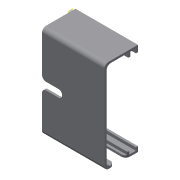
# Autodesk Inventor part: 09_Lid_Electronics
Saved by Autodesk Inventor 2019.4 (Build 234330000, 330)
## iProperties
Created: 2021-03-22
Part Number: 09_Lid_Electronics
Material: Generic
Document SubType Name: Modeling
Designer: diederichbenedict
Density: 1 g/cm^3
Appearance: Default
Author: diederichbenedict
Autodesk Inventor part; units mm, degrees
ref_plane "YZ Plane" through (0, 0, 0) normal (1, 0, 0) x (0, 1, 0)
ref_plane "XZ Plane" through (0, 0, 0) normal (0, 1, 0) x (-1, 0, 0)
ref_plane "Work Plane1" through (-120.5, -62.5, -4) normal (-1, 0, 0) x (0, 1, 0)
sketch "Sketch1" plane through (-120.5, -62.5, -4) normal (-1, 0, 0) x (0, 1, 0)
  line L0 (125, 2) -> (125, -4) projected
  line L1 (0, 2) -> (125, 2) projected
  line L2 (0, 2) -> (0, -4) projected
  line L3 (125, -4) -> (0, -4) projected
  line L4 (129, 6) -> (126, 6)
  line L5 (126, 6) -> (126, -42)
  line L6 (126, -42) -> (129, -42)
  line L7 (129, -42) -> (129, 6)
  line L8 (126, 6) -> (119.9159, 6)
  line L9 (119.9159, 6) -> (119.9159, 3)
  line L10 (119.9159, 3) -> (126, 3)
  line L11 (126, 3) -> (126, 6)
  line L12 (126, -5) -> (119.9159, -5)
  line L13 (119.9159, -5) -> (119.9159, -8)
  line L14 (119.9159, -8) -> (126, -8)
  line L15 (126, -8) -> (126, -5)
  line L16 (126, -42) -> (-4, -42)
  line L17 (-4, -42) -> (-4, -39)
  line L18 (-4, -39) -> (126, -39)
  line L19 (126, -39) -> (126, -42)
  line L20 (-4, -39) -> (-1, -39)
  line L21 (-1, -39) -> (-1, 6)
  line L22 (-1, 6) -> (-4, 6)
  line L23 (-4, 6) -> (-4, -39)
  line L24 (-4, 6) -> (3.1854, 6)
  line L25 (3.1854, 6) -> (3.1854, 3)
  line L26 (3.1854, 3) -> (-4, 3)
  line L27 (-4, 3) -> (-4, 6)
  line L28 (-1, -6.2816) -> (3.1854, -6.2816)
  line L29 (3.1854, -6.2816) -> (3.1854, -8.6145)
  line L30 (3.1854, -8.6145) -> (-1, -8.6145)
  line L31 (-1, -8.6145) -> (-1, -6.2816)
  point P0 (62.5, -4)
  dimension "d0" = 1
  dimension "d1" = 1
  dimension "d2" = 3
  dimension "d3" = 3
  dimension "d4" = 35
  dimension "d5" = 3
  dimension "d6" = 3
  dimension "d7" = 3
  dimension "d8" = 3
  dimension "d10" = 1
  dimension "d11" = 1
  dimension "d12" = 1
  constraints: 56 end point, 14 parallel, 7 horizontal, 7 perpendicular, 6 point on line
  measures "d0" distance between parallel lines of L21 L2
  measures "d1" distance between parallel lines of L26 L1
  measures "d2" distance between parallel lines of L26 L24
  measures "d3" distance between parallel lines of L23 L21
  measures "d4" distance between parallel lines of L3 L18
  measures "d5" distance between parallel lines of L18 L16
  measures "d6" distance between parallel lines of L5 L7
  measures "d7" distance between parallel lines of L14 L12
  measures "d8" distance between parallel lines of L10 L8
  measures "d10" distance between parallel lines of L1 L10
  measures "d11" distance between parallel lines of L12 L3
  measures "d12" distance between parallel lines of L5 L0
ref_plane "Work Plane2" through (-30.8635, -34.8198, 0.8246) normal (1, 0, 0) x (0, 1, 0)
extrude "Extrusion1" add sketch "Sketch1" against normal up to surface (89.6365 mm away) contours L7 L6 L5 L4 | L5 L10 L9 L8 | L16 L17 L18 L5 | L5 L14 L13 L12 | L18 L23 L26 L21 | L21 L28 L29 L30 | L23 L22 L21 L26 | L21 L24 L25 L26
fillet "Fillet1" radius 6 4 edges at (-75.6817, 66.5, 38) (-75.6817, -63.5, 35) (-75.6817, -66.5, 38) (-75.6817, 63.5, 35)
sketch "Sketch2" plane through (-120.5, -60.5, 38) normal (0, 0, 1) x (1, 0, 0)
  circle A0 centre (5, 57.8236) radius 3.5 projected
  line L0 (-37.6533, 57.8236) -> (23.6228, 57.8236) construction
  line L1 (-37.6533, 52.5159) -> (23.6228, 52.5159)
  line L2 (23.6228, 63.1312) -> (-37.6533, 63.1312)
  arc A1 (-37.6533, 63.1312) -> (-37.6533, 52.5159) centre (-37.6533, 57.8236) ccw
  arc A2 (23.6228, 52.5159) -> (23.6228, 63.1312) centre (23.6228, 57.8236) ccw
  point P0 (120.5, 60.5)
  point P1 (-7.0153, 57.8236)
  constraints: 8 end point, 4 point on circle, 4 tangent, 2 centre point, 1 horizontal, 1 midpoint, 1 parallel
extrude "Extrusion2" cut sketch "Sketch2" against normal through all contours A0 | A1 L2 A2 L1
sketch "Sketch3" plane through (-120.5, -66.5, -10) normal (0, -1, 0) x (1, 0, 0)
  line L0 (0, 42) -> (89.6365, 42) projected
  line L1 (0, 0) -> (0, 42) projected
  line L2 (0, 0) -> (89.6365, 0) projected
  line L3 (89.6365, 0) -> (89.6365, 42) projected
  line L4 (125.9655, 25.7695) -> (62.1359, 25.7695) construction
  line L5 (125.9655, 17.7908) -> (62.1359, 17.7908)
  line L6 (62.1359, 33.7482) -> (125.9655, 33.7482)
  arc A0 (125.9655, 17.7908) -> (125.9655, 33.7482) centre (125.9655, 25.7695) ccw
  arc A1 (62.1359, 33.7482) -> (62.1359, 17.7908) centre (62.1359, 25.7695) ccw
  point P0 (120.5, 10)
  point P1 (94.0507, 25.7695)
  constraints: 8 end point, 4 point on circle, 4 tangent, 2 centre point, 1 horizontal, 1 midpoint, 1 parallel
extrude "Extrusion3" cut sketch "Sketch3" against normal blind 10 contours L6 A0 L5 L3 | L3 L5 A1 L6
fillet "Fillet2" radius 6 4 edges at (-30.8635, -65, 23.7482) (-30.8635, -65, 7.7908) (-120.5, 2.6312, 36.5) (-120.5, -7.9841, 36.5)
body "Solid1"
